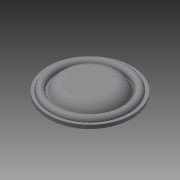
# Autodesk Inventor part: 2SS-LR
Saved by Autodesk Inventor 2014 SP2 (Build 180246200, 246)
## iProperties
Created: 2018-12-09
Part Number: 2SS-LR
Material: Generic
Catalog Web Link: www.cadenas.de
Description: 2 Series Stainless Steel Lower Race-Capacitiy up to 325 lbs Each
Vendor: COLSONGROUP
Document SubType Name: Modeling
Designer: psadmin
Manufacturer: COLSONGROUP
Mass: 8.1819 g
Surface Area: 59.0395 cm^2
Volume: 8.1819 cm^3
Density: 1 g/cm^3
Appearance: PSOLRGB-175-175-175
Category: PARTsolutions
Company: COLSONGROUP
Title: 2SS-LR
Author: Cadenas PARTsolutions
Comments: Capacitiy up to 325 lbs Each
PSOL_IDENT_0: {$CADENAS_DATA\23d-libs\colsongroup\colson\casters\2_series_stainless_steel\2_series_stainless_steel
PSOL_IDENT_1: _lower_race.prj},181 {VTYP=3D},{NB=2SS-LR},{LINA=2SS-LR},{NN=2 Series Stainless Steel Lower Race},{D
PSOL_IDENT_2: ATE=13.07.2017 07:15:59},{GEOMDATE=02.02.2017 09:18:26},{VERSION=},{LINEID=40},{WBVAR=},{WBNUMERIC=}
PSOL_IDENT_3: {NB=2SS-LR},{LINA=2SS-LR},{KT=DUMMY},{PN=2SS-LR}
NN: 2 Series Stainless Steel Lower Race
NT: Capacitiy up to 325 lbs Each
NB: 2SS-LR
NBSYN: $PN.
LINA: 2SS-LR
PN: 2SS-LR
SUPPLIER: COLSONGROUP
ARTICLENO: 2SS-LR
BOMINFO: 2SS-LR
CREATOR: CADENAS GmbH
Autodesk Inventor part; units mm, degrees
sketch "Sketch_1" plane through (0, 0, 0) normal (0, 0, 1) x (1, 0, 0)
  line L0 (0, -9.0932) -> (0, 0)
  line L1 (0, 0) -> (11.5316, 0)
  arc A0 (17.9105, -4.2968) -> (11.5316, 0) centre (11.5316, -6.8834) ccw
  arc A1 (17.9105, -4.2968) -> (24.1241, -4.8006) centre (21.1328, -3.1242) ccw
  line L2 (24.1241, -4.8006) -> (25.781, -4.8006)
  line L3 (25.781, -4.8006) -> (25.781, -6.869)
  arc A2 (15.6069, -5.3811) -> (25.781, -6.869) centre (21.1328, -3.1242) ccw
  arc A3 (15.6069, -5.3811) -> (11.5316, -2.54) centre (11.5316, -6.8834) ccw
  line L4 (11.5316, -2.54) -> (0, -2.54)
  line L5 (0, -2.54) -> (0, 0)
  constraints: 12 end point, 8 point on circle, 4 centre point
revolve "Revolution1" add sketch "Sketch_1" angle 360 about axis through (0, -9.0932, 0) along (0, -1, 0)
sketch "Sketch_2" plane through (0, 0, 0) normal (0, 0, 1) x (1, 0, 0)
  line L0 (0, -12.7) -> (0, 12.7)
  circle A0 centre (21.59, -4.826) radius 2.286
  constraints: 2 end point, 1 centre point
revolve "Revolution2" add sketch "Sketch_2" angle 360 about axis through (0, -12.7, 0) along (0, -1, 0)
ref_plane "lower_race_XY" through (0, 0, 0) normal (0, -1, 0) x (1, 0, 0)
ref_plane "lower_race_YZ" through (0, 0, 0) normal (1, 0, 0) x (0, 0, 1)
ref_plane "lower_race_ZX" through (0, 0, 0) normal (0, 0, 1) x (0, -1, 0)
body "Solid1"
